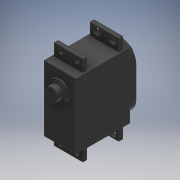
# Autodesk Inventor part: krs2350_hv_sa
Saved by Autodesk Inventor 2018 (Build 220112000, 112)
## iProperties
Created: 2018-07-05
Part Number: krs2350_hv_sa
Material: 一般
Document SubType Name: Modeling
Designer: shun
Density: 1 g/cm^3
Appearance: 滑らか - 黒
Mass: 32.2184 g
Surface Area: 76.9749 cm^2
Volume: 32.2184 cm^3
Author: shun
Autodesk Inventor part; units mm, degrees
sketch "スケッチ1" plane through (0, 0, 0) normal (0, 1, 0) x (-1, 0, 0)
  circle A0 centre (0, 0) radius 3
  dimension "d0" = 6
  constraints: 1 centre point, 1 coincident
  measures "d0" diameter of A0
extrude "押し出し1" add sketch "スケッチ1" along normal blind 5.2
sketch "スケッチ2" plane through (0, 0, 0) normal (0, -1, 0) x (1, 0, 0)
  circle A0 centre (0, 0) radius 10
  dimension "d3" = 20
  constraints: 1 centre point, 1 coincident
  measures "d3" diameter of A0
extrude "押し出し2" add sketch "スケッチ2" along normal blind 4
sketch "スケッチ3" plane through (0, -4, 0) normal (0, -1, 0) x (1, 0, 0)
  line L0 (0, 0) -> (0, -9.6) construction
  line L1 (10, 10.9) -> (-10, 10.9)
  line L2 (-10, 10.9) -> (-10, -30.1)
  line L3 (-10, -30.1) -> (10, -30.1)
  line L4 (10, -30.1) -> (10, 10.9)
  line L5 (10, 10.9) -> (-10, -30.1) construction
  line L6 (-10, 10.9) -> (10, -30.1) construction
  dimension "d6" = 9.6
  dimension "d7" = 20
  dimension "d8" = 41
  constraints: 14 end point, 2 midpoint, 2 parallel, 1 horizontal, 1 perpendicular, 1 vertical
  measures "d6" distance of L0.start L0.end
  measures "d7" distance of L3.end L2.end
  measures "d8" distance of L2.end L1.end
extrude "押し出し3" add sketch "スケッチ3" along normal blind 33.8
sketch "スケッチ4" plane through (0, -4, 0) normal (0, 1, 0) x (1, 0, 0)
  circle A0 centre (0, 0) radius 3 construction
  line L0 (0, 0) -> (0, 19.2) construction
  arc A1 (10, 19.2) -> (-10, 19.2) centre (0, 19.2) ccw
  line L1 (-10, 19.2) -> (-10, 0)
  circle A2 centre (0, 0) radius 10 construction
  line L2 (10, 19.2) -> (10, 0)
  line L3 (10, 30.1) -> (10, -10.9) projected
  arc A3 (10, 0) -> (-10, 0) centre (0, 0) ccw
  dimension "d11" = 19.2
  dimension "d12" = 10
  constraints: 6 end point, 4 point on circle, 4 vertical, 2 centre point, 2 coincident, 1 horizontal alignment, 1 point on line, 1 other
  measures "d11" distance of L0.start L0.end
  measures "d12" radius of A1
extrude "押し出し4" add sketch "スケッチ4" along normal blind 4
ref_plane "作業平面1" through (0, 1.3, 0) normal (0, 1, 0) x (1, 0, 0)
sketch "スケッチ5" plane through (0, 0, 0) normal (0, 1, 0) x (1, 0, 0)
  circle A0 centre (0, 0) radius 6.25
  dimension "d16" = 12.5
  constraints: 1 centre point, 1 coincident
  measures "d16" diameter of A0
sketch "スケッチ6" plane through (0, 1.3, 0) normal (0, 1, 0) x (1, 0, 0)
  circle A0 centre (0, 0) radius 5.5
  dimension "d17" = 11
  constraints: 1 centre point, 1 coincident
  measures "d17" diameter of A0
loft "ロフト1" add profiles "スケッチ5", "スケッチ6"
ref_plane "作業平面2" through (0, -9.9, 0) normal (0, 1, 0) x (1, 0, 0)
ref_plane "作業平面3" through (0, -29.9, 0) normal (0, -1, 0) x (1, 0, 0)
sketch "スケッチ7" plane through (0, -9.9, 0) normal (0, 1, 0) x (1, 0, 0)
  line L0 (10, -10.9) -> (-10, -10.9) projected
  line L1 (9, -10.9) -> (-9, -10.9)
  line L2 (-9, -10.9) -> (-9, -18.4)
  line L3 (-9, -18.4) -> (9, -18.4)
  line L4 (9, -18.4) -> (9, -10.9)
  line L5 (10, 30.1) -> (10, -10.9) projected
  line L6 (9, -15.4) -> (-9, -15.4) construction
  circle A0 centre (5, -15.4) radius 2.35
  circle A1 centre (-5, -15.4) radius 2.35
  point P0 (0, 0)
  dimension "d24" = 18
  dimension "d25" = 7.5
  dimension "d26" = 1
  dimension "d27" = 3
  dimension "d28" = 4.7
  dimension "d29" = 4
  dimension "d30" = 4.7
  dimension "d31" = 4
  constraints: 10 end point, 5 point on line, 2 centre point, 2 parallel, 2 perpendicular, 1 horizontal
  measures "d24" distance of L3.end L2.end
  measures "d25" distance of L2.end L1.end
  measures "d26" distance between parallel lines of L5 L4
  measures "d27" distance between parallel lines of L3 L6
  measures "d28" diameter of A0
  measures "d29" distance from line of L4 A0.centre
  measures "d30" diameter of A1
  measures "d31" distance from line of L2 A1.centre
extrude "押し出し5" add sketch "スケッチ7" along normal blind 2.5
ref_plane "作業平面4" through (10, -4, -9.6) normal (0, 0, -1) x (-1, 0, 0)
mirror "ミラー1" about plane through (10, -4, -9.6) normal (0, 0, -1) of "押し出し5"
sketch "スケッチ8" plane through (0, -29.9, 0) normal (0, -1, 0) x (1, 0, 0)
  line L0 (10, 10.9) -> (-10, 10.9) projected
  line L1 (9, 10.9) -> (-9, 10.9)
  line L2 (-9, 10.9) -> (-9, 18.4)
  line L3 (-9, 18.4) -> (9, 18.4)
  line L4 (9, 18.4) -> (9, 10.9)
  line L5 (10, -30.1) -> (10, 10.9) projected
  line L6 (9, 18.4) -> (9, 10.9) projected
  line L7 (9, 15.4) -> (-9, 15.4) construction
  line L8 (-9, 10.9) -> (-9, 18.4) projected
  circle A0 centre (5, 15.4) radius 1.6
  circle A1 centre (-5, 15.4) radius 1.6
  point P0 (0, 0)
  dimension "d35" = 18
  dimension "d36" = 7.5
  dimension "d37" = 1
  dimension "d38" = 3
  dimension "d39" = 3.2
  dimension "d40" = 4
  dimension "d41" = 3.2
  dimension "d42" = 4
  constraints: 10 end point, 5 point on line, 2 centre point, 2 parallel, 2 perpendicular, 1 horizontal
  measures "d35" distance of L2.end L3.end
  measures "d36" distance of L1.end L2.end
  measures "d37" distance between parallel lines of L4 L5
  measures "d38" distance between parallel lines of L3 L7
  measures "d39" diameter of A0
  measures "d40" distance from line of L4 A0.centre
  measures "d41" diameter of A1
  measures "d42" distance from line of L2 A1.centre
extrude "押し出し6" add sketch "スケッチ8" along normal blind 2.5
mirror "ミラー2" about plane through (10, -4, -9.6) normal (0, 0, -1) of "押し出し6"
sketch "スケッチ9" plane through (0, -37.8, 0) normal (0, -1, 0) x (1, 0, 0)
  circle A0 centre (0, 0) radius 4
  dimension "d45" = 8
  constraints: 1 centre point, 1 coincident
  measures "d45" diameter of A0
extrude "押し出し7" add sketch "スケッチ9" along normal blind 5.3
sketch "スケッチ10" plane through (0, -37.8, 0) normal (0, -1, 0) x (1, 0, 0)
  circle A0 centre (0, 0) radius 6
  dimension "d48" = 12
  constraints: 1 centre point, 1 coincident
  measures "d48" diameter of A0
extrude "押し出し8" add sketch "スケッチ10" along normal blind 1.3
sketch "スケッチ11" plane through (0, -39.1, 0) normal (0, -1, 0) x (1, 0, 0)
  circle A0 centre (0, 0) radius 5
  dimension "d51" = 10
  constraints: 1 centre point, 1 coincident
  measures "d51" diameter of A0
extrude "押し出し9" add sketch "スケッチ11" along normal blind 0.5
